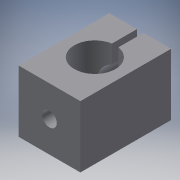
# Autodesk Inventor part: 22-134 Block
Saved by Autodesk Inventor 2018 (Build 220105000, 105)
## iProperties
Created: 2004-11-24
Part Number: 22-134 Block
Document SubType Name: Modeling
Designer: Autodesk, Inc.
Manufacturer: Standard
Standards Organization: Custom
Description: SLIDE COLLAR BLOCK
Mass: 55.6668 g
Surface Area: 149.462 cm^2
Volume: 55.6668 cm^3
Density: 1 g/cm^3
Material: Generic
Appearance: Default
CAGE: 1LJX3
Dept. ID: Product Design
Description #2: ---
Finish #1: ---
Finish #2: ---
Material ID: ---
Project Number: ---
Author: Autodesk, Inc.
Autodesk Inventor part; units mm, degrees
ref_plane "YZ Plane" through (0, 0, 0) normal (1, 0, 0) x (0, 1, 0)
ref_plane "XZ Plane" through (0, 0, 0) normal (0, 1, 0) x (-1, 0, 0)
sketch "Sketch1" plane through (0, 0, 0) normal (0, 0, 1) x (1, 0, 0)
  line L0 (-19.05, 19.05) -> (19.05, 19.05)
  line L1 (19.05, 19.05) -> (19.05, -19.05)
  line L2 (19.05, -19.05) -> (-19.05, -19.05)
  line L3 (-19.05, -19.05) -> (-19.05, 19.05)
  point P0 (0, 0)
  point P1 (-19.05, 0)
  point P2 (0, 19.05)
  dimension "d0" = 38.1
  constraints: 8 end point, 2 midpoint, 2 parallel, 2 perpendicular, 1 horizontal, 1 horizontal alignment, 1 vertical alignment
  measures "d0" distance of L0.start L0.end
extrude "Extrusion1" add sketch "Sketch1" along normal blind 56
sketch "Sketch2" plane through (-19.05, 19.05, 0) normal (0, 1, 0) x (1, 0, 0)
  circle A0 centre (19.05, -28) radius 12.7
  line L0 (0, 0) -> (38.1, 0) projected
  line L1 (0, -56) -> (38.1, -56) projected
  line L2 (17.05, 0) -> (21.05, 0)
  line L3 (21.05, 0) -> (21.05, -28)
  line L4 (21.05, -28) -> (17.05, -28)
  line L5 (17.05, -28) -> (17.05, 0)
  point P0 (19.05, 0)
  dimension "d3" = 28
  dimension "d4" = 25.4
  dimension "d5" = 4
  constraints: 8 end point, 3 midpoint, 2 parallel, 1 centre point, 1 coincident, 1 horizontal, 1 perpendicular, 1 point on line, 1 vertical alignment
  measures "d3" distance from line of A0.centre L1
  measures "d4" diameter of A0
  measures "d5" distance between parallel lines of L3 L5
extrude "Extrusion2" cut sketch "Sketch2" against normal through all
ref_plane "Work Plane1" through (0, 0, 48) normal (0, 0, 1) x (1, 0, 0)
sketch "Sketch3" plane through (0, 0, 48) normal (0, 0, 1) x (1, 0, 0)
  point P0 (0, 0)
hole "Hole1" at (0, 0, 48) direction (0, 0, 1) diameter 9 end through all clearance for "Flat Head Machine Screw" size "M8" standard "Ansi Metric M Profile"
sketch "Sketch4" plane through (0, 0, 0) normal (0, 0, -1) x (-1, 0, 0)
  circle A0 centre (0, 0) radius 8
  dimension "d16" = 16
  constraints: 1 centre point, 1 coincident
  measures "d16" diameter of A0
extrude "Extrusion3" cut sketch "Sketch4" against normal up to surface (48 mm away)
sketch "Sketch5" plane through (-19.05, -19.05, 0) normal (-1, 0, 0) x (0, 0, 1)
  line L0 (0, 0) -> (0, 38.1) projected
  circle A0 centre (5.7121, 19.05) radius 3.8228
  line L1 (4.9053, 27.6435) -> (6.5597, 27.6435)
  line L2 (6.5597, 27.6435) -> (6.5597, 10.4565)
  line L3 (6.5597, 10.4565) -> (4.9053, 10.4565)
  line L4 (4.9053, 10.4565) -> (4.9053, 27.6435)
  point P0 (0, 19.05)
  point P1 (6.5597, 19.05)
  constraints: 8 end point, 2 horizontal alignment, 2 midpoint, 2 parallel, 1 centre point, 1 horizontal, 1 perpendicular
extrude "Extrusion4" add sketch "Sketch5" along normal blind 6
body "Solid1"
